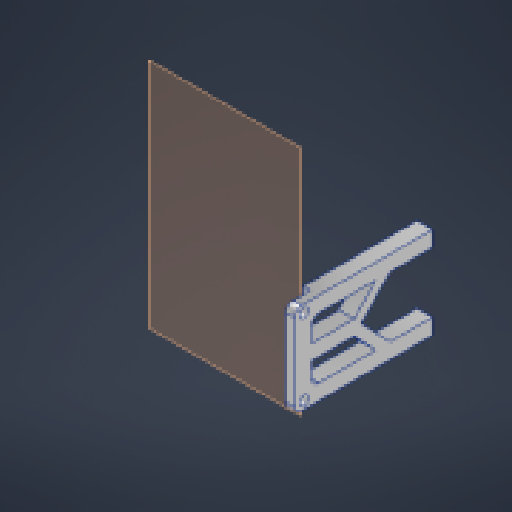
# Autodesk Inventor part: 106_64_Connector
Saved by Autodesk Inventor 2024 (Build 280153000, 153)
## iProperties
Created: 2024-01-23
Part Number: 106_64_Connector
Material: 알루미늄 6061
Document SubType Name: Modeling
Designer: ASUS
Density: 2.7 g/cm^3
Appearance: 알루미늄 - 평지
Author: ASUS
Autodesk Inventor part; units mm, degrees
ref_plane "YZ Plane" through (0, 0, 0) normal (1, 0, 0) x (0, 1, 0)
ref_plane "XZ Plane" through (0, 0, 0) normal (0, 1, 0) x (-1, 0, 0)
ref_plane "XY Plane" through (0, 0, 0) normal (0, 0, 1) x (1, 0, 0)
ref_plane "작업 평면1" through (-20.6428, -10.415, 0) normal (0, 0, 1) x (1, 0, 0)
sketch "스케치1" plane through (-20.6428, -10.415, 0) normal (0, 0, 1) x (1, 0, 0)
  arc A0 (40.7428, 14.9916) -> (40.2236, 16.6785) centre (37.7428, 14.9916) ccw projected
  line L0 (40.2236, 16.6785) -> (36.2381, 22.5396) projected
  arc A1 (36.2381, 22.5396) -> (34.5842, 23.415) centre (34.5842, 21.415) ccw projected
  line L1 (33.6428, 23.415) -> (34.5842, 23.415) projected
  arc A2 (35.1428, 21.915) -> (33.6428, 23.415) centre (33.6428, 21.915) ccw projected
  line L2 (35.1428, -31.085) -> (35.1428, 21.915) projected
  arc A3 (34.1428, -32.085) -> (35.1428, -31.085) centre (34.1428, -31.085) ccw projected
  line L3 (7.1428, -32.085) -> (34.1428, -32.085) projected
  arc A4 (6.1428, -31.085) -> (7.1428, -32.085) centre (7.1428, -31.085) ccw projected
  line L4 (6.1428, 21.915) -> (6.1428, -31.085) projected
  arc A5 (7.6428, 23.415) -> (6.1428, 21.915) centre (7.6428, 21.915) ccw projected
  line L5 (6.7014, 23.415) -> (7.6428, 23.415) projected
  arc A6 (6.7014, 23.415) -> (5.0476, 22.5396) centre (6.7014, 21.415) ccw projected
  line L6 (5.0476, 22.5396) -> (1.0621, 16.6785) projected
  arc A7 (1.0621, 16.6785) -> (0.5428, 14.9916) centre (3.5428, 14.9916) ccw projected
  line L7 (0.5428, 14.9916) -> (0.5428, -29.2617) projected
  arc A8 (0.5428, -29.2617) -> (1.0621, -30.9486) centre (3.5428, -29.2617) ccw projected
  line L8 (1.0621, -30.9486) -> (4.7499, -36.372) projected
  arc A9 (4.7499, -36.372) -> (7.2307, -37.685) centre (7.2307, -34.685) ccw projected
  line L9 (7.2307, -37.685) -> (34.0549, -37.685) projected
  arc A10 (34.0549, -37.685) -> (36.5357, -36.372) centre (34.0549, -34.685) ccw projected
  line L10 (36.5357, -36.372) -> (40.2236, -30.9486) projected
  arc A11 (40.2236, -30.9486) -> (40.7428, -29.2617) centre (37.7428, -29.2617) ccw projected
  line L11 (40.7428, -29.2617) -> (40.7428, 14.9916) projected
  circle A12 centre (3.3428, 14.415) radius 1.35 projected
  circle A13 centre (3.3428, -7.585) radius 1.35 projected
  circle A14 centre (9.6428, -34.885) radius 1.35 projected
  circle A15 centre (37.9428, 14.415) radius 1.35 projected
  circle A16 centre (37.9428, -7.585) radius 1.35 projected
  circle A17 centre (31.6428, -34.885) radius 1.35 projected
  circle A18 centre (3.3428, -29.585) radius 1.35 projected
  circle A19 centre (37.9428, -29.585) radius 1.35 projected
  line L12 (35.6928, -9.835) -> (40.1928, -9.835)
  line L13 (40.1928, -9.835) -> (40.1928, -5.335)
  line L14 (40.1928, -5.335) -> (35.6928, -5.335)
  line L15 (35.6928, -5.335) -> (35.6928, -9.835)
  line L16 (35.6928, -9.835) -> (40.1928, -5.335) construction
  line L17 (40.1928, -9.835) -> (35.6928, -5.335) construction
  line L18 (35.6928, -31.835) -> (40.1928, -31.835)
  line L19 (40.1928, -31.835) -> (40.1928, -27.335)
  line L20 (40.1928, -27.335) -> (35.6928, -27.335)
  line L21 (35.6928, -27.335) -> (35.6928, -31.835)
  line L22 (35.6928, -31.835) -> (40.1928, -27.335) construction
  line L23 (40.1928, -31.835) -> (35.6928, -27.335) construction
  point P0 (20.6428, 10.415)
  dimension "d0" = 4.5
  dimension "d1" = 4.5
  dimension "d2" = 4.5
  dimension "d3" = 4.5
  constraints: 24 end point, 4 midpoint, 4 parallel, 2 horizontal, 2 perpendicular
  measures "d0" distance of L14.end L13.end
  measures "d1" distance of L13.end L12.end
  measures "d2" distance of L20.end L19.end
  measures "d3" distance of L19.end L18.end
extrude "돌출1" add sketch "스케치1" along normal blind 20 contours L19 L18 L10 | L10 L18 L21 L20 L19 | A16 | A19 | L15 L14 L13 L12
sketch "스케치2" plane through (19.55, -42.25, 0) normal (1, 0, 0) x (0, 0, -1)
  line L0 (0, 0) -> (0, 4.5) projected
  line L1 (0, 4.5) -> (-20, 4.5) projected
  line L2 (-20, 0) -> (-20, 4.5) projected
  line L3 (0, 0) -> (-20, 0) projected
  line L4 (0, 22) -> (0, 26.5) projected
  line L5 (0, 26.5) -> (-20, 26.5) projected
  line L6 (-20, 22) -> (-20, 26.5) projected
  line L7 (0, 22) -> (-20, 22) projected
  line L8 (-20, 0) -> (-20, 26.5)
  line L9 (-20, 26.5) -> (-15, 26.5)
  line L10 (-15, 26.5) -> (-15, 0)
  line L11 (-15, 0) -> (-20, 0)
  point P0 (0, 42.25)
  point P1 (-15, 4.5)
  point P2 (-15, 22)
  point P3 (-20, 22)
  point P4 (-20, 4.5)
  dimension "d6" = 5
  constraints: 8 end point, 2 parallel, 1 collinear, 1 perpendicular
  measures "d6" distance of L5.end L9.end
extrude "돌출2" add sketch "스케치2" against normal up to surface (4.5 mm away) contours L1 L8 L7 L10
fillet "모깎기1" radius 2 2 edges at (17.3, -20.25, 15) (17.3, -37.75, 15)
fillet "모깎기2" radius 2 2 edges at (17.3, -42.25, 20) (17.3, -15.75, 20)
sketch "스케치3" plane through (-20.6428, -10.415, 0) normal (0, 0, -1) x (-1, 0, 0)
  circle A0 centre (-37.9428, -29.585) radius 1.35 projected
  circle A1 centre (-37.9428, -7.585) radius 1.35 projected
  circle A2 centre (-37.9428, -29.585) radius 1.05
  circle A3 centre (-37.9428, -7.585) radius 1.05
  point P0 (-20.6428, 10.415)
  dimension "d11" = 2.1
  dimension "d12" = 2.1
  constraints: 2 centre point, 2 coincident
  measures "d11" diameter of A2
  measures "d12" diameter of A3
extrude "돌출3" cut sketch "스케치3" against normal blind 10 contours A2 | A3
sketch "스케치4" plane through (15.05, -15.75, 0) normal (0, 1, 0) x (1, 0, 0)
  line L0 (4.5, -18) -> (0, -18) projected
  line L1 (-30.1, -18) -> (-34.6, -18)
  line L2 (0, 0) -> (0, -18) projected
  line L3 (0, -18) -> (-30.1, -18)
  line L4 (2.05, -13) -> (-32.15, -13)
  line L5 (-32.15, -13) -> (-32.15, -23)
  line L6 (-32.15, -23) -> (2.05, -23)
  line L7 (2.05, -23) -> (2.05, -13)
  line L8 (2.05, -13) -> (-32.15, -23) construction
  line L9 (-32.15, -13) -> (2.05, -23) construction
  point P0 (-15.05, 0)
  point P1 (-15.05, -18)
  dimension "d15" = 34.2
  dimension "d16" = 10
  constraints: 16 end point, 3 midpoint, 2 horizontal, 2 parallel, 2 perpendicular, 2 other
  measures "d15" distance of L6.end L5.end
  measures "d16" distance of L5.end L4.end
extrude "돌출4" cut sketch "스케치4" against normal up to surface (26.5 mm away)
sketch "스케치5" plane through (19.55, -42.25, 0) normal (1, 0, 0) x (0, 0, -1)
  circle A0 centre (-17.3, 2.25) radius 1.35
  circle A1 centre (-17.3, 24.25) radius 1.35
  point P0 (0, 42.25)
  constraints: 2 centre point, 4 other
extrude "돌출5" cut sketch "스케치5" against normal through all
sketch "스케치6" plane through (-20.6428, -10.415, 0) normal (0, 0, -1) x (-1, 0, 0)
  circle A0 centre (-37.9428, -29.585) radius 1.05 projected
  line L0 (-35.6928, -31.835) -> (-40.1928, -31.835) projected
  line L1 (-35.6928, -27.335) -> (-35.6928, -31.835) projected
  line L2 (-40.1928, -27.335) -> (-35.6928, -27.335) projected
  line L3 (-40.1928, -31.835) -> (-40.1928, -27.335) projected
  circle A1 centre (-37.9428, -7.585) radius 1.05 projected
  line L4 (-40.1928, -9.835) -> (-40.1928, -5.335) projected
  line L5 (-35.6928, -9.835) -> (-40.1928, -9.835) projected
  line L6 (-35.6928, -5.335) -> (-35.6928, -9.835) projected
  line L7 (-40.1928, -5.335) -> (-35.6928, -5.335) projected
  point P0 (-20.6428, 10.415)
extrude "돌출6" add sketch "스케치6" along normal blind 20
sketch "스케치7" plane through (19.55, -35.75, 15) normal (1, 0, 0) x (0, 0, -1)
  circle A0 centre (-2.3, 17.75) radius 1.35 projected
  circle A1 centre (-2.3, -4.25) radius 1.35 projected
  arc A2 (-3, 20) -> (-5, 18) centre (-3, 18) ccw projected
  line L0 (-5, -4.5) -> (-5, 18) projected
  arc A3 (-5, -4.5) -> (-3, -6.5) centre (-3, -4.5) ccw projected
  line L1 (35, -6.5) -> (-3, -6.5) projected
  line L2 (35, -2) -> (35, -6.5) projected
  line L3 (35, -2) -> (2, -2) projected
  arc A4 (0, 0) -> (2, -2) centre (2, 0) ccw projected
  line L4 (0, 0) -> (0, 13.5) projected
  arc A5 (2, 15.5) -> (0, 13.5) centre (2, 13.5) ccw projected
  line L5 (2, 15.5) -> (35, 15.5) projected
  line L6 (35, 20) -> (35, 15.5) projected
  line L7 (35, 20) -> (-3, 20) projected
  circle A6 centre (-2.3, 17.75) radius 1.35 projected
  circle A7 centre (-2.3, -4.25) radius 1.35 projected
  arc A8 (0, 0) -> (2, -2) centre (2, 0) ccw projected
  line L8 (2, -2) -> (2, -6.5) projected
  line L9 (-3, -6.5) -> (2, -6.5) projected
  arc A9 (-5, -4.5) -> (-3, -6.5) centre (-3, -4.5) ccw projected
  line L10 (-5, 18) -> (-5, -4.5) projected
  arc A10 (-3, 20) -> (-5, 18) centre (-3, 18) ccw projected
  line L11 (2, 20) -> (-3, 20) projected
  line L12 (2, 20) -> (2, 15.5) projected
  arc A11 (2, 15.5) -> (0, 13.5) centre (2, 13.5) ccw projected
  line L13 (0, 0) -> (0, 13.5) projected
  line L14 (2, -2) -> (18.5, 15.5)
  line L15 (6.1232, -2) -> (22.6232, 15.5)
  line L16 (2, 15.5) -> (18.5, -2)
  line L17 (6.1232, 15.5) -> (22.6232, -2)
  line L18 (12.3116, 4.5635) -> (12.3116, 8.9365)
  line L19 (12.3116, 8.9365) -> (0, 8.9365)
  line L20 (0, 8.9365) -> (0, 4.5635)
  line L21 (0, 4.5635) -> (12.3116, 4.5635)
  point P0 (15, 35.75)
  point P1 (14.3732, 6.75)
  point P2 (0, 8.9365)
  dimension "d23" = 3
  dimension "d24" = 3
  constraints: 16 end point, 8 point on line, 4 parallel, 2 midpoint, 1 perpendicular
  measures "d23" distance between parallel lines of L14 L15
  measures "d24" distance between parallel lines of L16 L17
extrude "돌출7" add sketch "스케치7" against normal up to surface (4.5 mm away) contours L19 L14 L16 | L16 L14 L21 L4 L19 | L15 L17 L14 L5 | L18 L16 L14 | L17 L15 L18 | L16 L21 L14 | L17 L3 L16 L15
sketch "스케치8" plane through (17.1, -15.75, 13) normal (-1, 0, 0) x (0, 0, 1)
  circle A0 centre (4.3, -2.25) radius 1.35 projected
  circle A1 centre (4.3, -24.25) radius 1.35 projected
  arc A2 (0, -22) -> (2, -20) centre (0, -20) ccw projected
  line L0 (0, -22) -> (0, -26.5) projected
  line L1 (5, -26.5) -> (0, -26.5) projected
  arc A3 (5, -26.5) -> (7, -24.5) centre (5, -24.5) ccw projected
  line L2 (7, -2) -> (7, -24.5) projected
  arc A4 (7, -2) -> (5, 0) centre (5, -2) ccw projected
  line L3 (0, 0) -> (5, 0) projected
  line L4 (0, 0) -> (0, -4.5) projected
  arc A5 (2, -6.5) -> (0, -4.5) centre (0, -6.5) ccw projected
  line L5 (2, -11.0635) -> (2, -6.5) projected
  line L6 (2, -15.4365) -> (2, -11.0635) projected
  line L7 (2, -20) -> (2, -15.4365) projected
  line L8 (0, -26.5) -> (0, -22) projected
  line L9 (-16.5, -22) -> (0, -22) projected
  line L10 (-10.3116, -15.4365) -> (-16.5, -22) projected
  line L11 (2, -15.4365) -> (-10.3116, -15.4365) projected
  line L12 (2, -11.0635) -> (2, -15.4365) projected
  line L13 (-10.3116, -11.0635) -> (2, -11.0635) projected
  line L14 (-16.5, -4.5) -> (-10.3116, -11.0635) projected
  line L15 (-16.5, -4.5) -> (0, -4.5) projected
  line L16 (0, -4.5) -> (0, 0) projected
  line L17 (-33, 0) -> (0, 0) projected
  line L18 (-33, -4.5) -> (-33, 0) projected
  line L19 (-33, -4.5) -> (-20.6232, -4.5) projected
  line L20 (-12.3732, -13.25) -> (-20.6232, -4.5) projected
  line L21 (-20.6232, -22) -> (-12.3732, -13.25) projected
  line L22 (-33, -22) -> (-20.6232, -22) projected
  line L23 (-33, -26.5) -> (-33, -22) projected
  line L24 (0, -26.5) -> (-33, -26.5) projected
  line L25 (-16.5, -4.5) -> (0, -4.5) projected
  line L26 (0, -4.5) -> (0, -22)
  point P0 (-13, 15.75)
  point P1 (0, -11.0635)
  point P2 (0, -15.4365)
  constraints: 2 end point, 1 perpendicular
extrude "돌출8" cut sketch "스케치8" along normal up to surface (2.05 mm away) contours L26 L13 L6 L11
